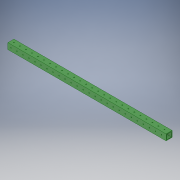
# Autodesk Inventor part: numbah 9
Saved by Autodesk Inventor 2018.2 (Build 222227000, 227)
## iProperties
Created: 2018-02-03
Part Number: numbah 9
Material: Generic
Document SubType Name: Modeling
Designer: matuch.michael
Density: 1 g/cm^3
Appearance: Smooth - Dark Forest Green
Author: matuch.michael
Autodesk Inventor part; units mm, degrees
ref_plane "YZ Plane" through (0, 0, 0) normal (1, 0, 0) x (0, 1, 0)
ref_plane "XZ Plane" through (0, 0, 0) normal (0, 1, 0) x (-1, 0, 0)
ref_plane "XY Plane" through (0, 0, 0) normal (0, 0, 1) x (1, 0, 0)
sketch "Sketch1" plane through (0, 0, 0) normal (0, 0, 1) x (1, 0, 0)
  line L0 (-12.5902, 5.4476) -> (654.49, 5.4476)
  line L1 (654.49, 5.4476) -> (654.49, -19.9524)
  line L2 (654.49, -19.9524) -> (-12.5902, -19.9524)
  line L3 (-12.5902, -19.9524) -> (-12.5902, 5.4476)
  point P0 (0, 0)
  dimension "d0" = 667.0802
  dimension "d1" = 25.4
  constraints: 8 end point, 2 parallel, 1 horizontal, 1 perpendicular
  measures "d0" distance of L1.end L2.end
  measures "d1" distance of L0.end L1.end
extrude "Extrusion1" add sketch "Sketch1" along normal blind 25.4
sketch "Sketch2" plane through (0, 0, 25.4) normal (0, 0, 1) x (1, 0, 0)
  circle A0 centre (0.1098, -7.2524) radius 1.9685
  line L0 (-12.5902, 5.4476) -> (-12.5902, -19.9524) projected
  line L1 (-12.5902, -19.9524) -> (654.49, -19.9524) projected
  circle A1 centre (25.5098, -7.2524) radius 1.9685
  circle A2 centre (50.9098, -7.2524) radius 1.9685
  circle A3 centre (76.3098, -7.2524) radius 1.9685
  circle A4 centre (101.7098, -7.2524) radius 1.9685
  circle A5 centre (127.1098, -7.2524) radius 1.9685
  circle A6 centre (152.5098, -7.2524) radius 1.9685
  circle A7 centre (177.9098, -7.2524) radius 1.9685
  circle A8 centre (203.3098, -7.2524) radius 1.9685
  circle A9 centre (228.7098, -7.2524) radius 1.9685
  circle A10 centre (254.1098, -7.2524) radius 1.9685
  circle A11 centre (279.5098, -7.2524) radius 1.9685
  circle A12 centre (304.9098, -7.2524) radius 1.9685
  circle A13 centre (330.3098, -7.2524) radius 1.9685
  circle A14 centre (355.7098, -7.2524) radius 1.9685
  circle A15 centre (381.1098, -7.2524) radius 1.9685
  circle A16 centre (406.5098, -7.2524) radius 1.9685
  circle A17 centre (431.9098, -7.2524) radius 1.9685
  circle A18 centre (457.3098, -7.2524) radius 1.9685
  circle A19 centre (482.7098, -7.2524) radius 1.9685
  circle A20 centre (508.1098, -7.2524) radius 1.9685
  circle A21 centre (533.5098, -7.2524) radius 1.9685
  circle A22 centre (558.9098, -7.2524) radius 1.9685
  circle A23 centre (584.3098, -7.2524) radius 1.9685
  circle A24 centre (609.7098, -7.2524) radius 1.9685
  circle A25 centre (635.1098, -7.2524) radius 1.9685
  circle A26 centre (635.1098, -7.2524) radius 1.9685
  circle A27 centre (660.5098, -7.2524) radius 1.9685
  circle A28 centre (685.9098, -7.2524) radius 1.9685
  point P0 (0, 0)
  dimension "d4" = 3.937
  dimension "d5" = 12.7
  dimension "d6" = 12.7
  dimension "d9" = 25.4
  dimension "d16" = 25.4
  constraints: 29 centre point, 2 horizontal, 56 other
  measures "d4" diameter of A0
  measures "d5" distance from line of L0 A0.centre
  measures "d6" distance from line of L1 A0.centre
  measures "d9" distance of A0.centre A1.centre
  measures "d16" distance of A24.centre A25.centre
sketch "Sketch4" plane through (-12.5902, 5.4476, 0) normal (0, 1, 0) x (1, 0, 0)
  circle A0 centre (12.7, -12.7) radius 1.9685
  line L0 (0, 0) -> (0, -25.4) projected
  line L1 (667.0802, -25.4) -> (0, -25.4) projected
  circle A1 centre (38.1, -12.7) radius 1.9685
  circle A2 centre (63.5, -12.7) radius 1.9685
  circle A3 centre (88.9, -12.7) radius 1.9685
  circle A4 centre (114.3, -12.7) radius 1.9685
  circle A5 centre (139.7, -12.7) radius 1.9685
  circle A6 centre (165.1, -12.7) radius 1.9685
  circle A7 centre (190.5, -12.7) radius 1.9685
  circle A8 centre (215.9, -12.7) radius 1.9685
  circle A9 centre (241.3, -12.7) radius 1.9685
  circle A10 centre (266.7, -12.7) radius 1.9685
  circle A11 centre (292.1, -12.7) radius 1.9685
  circle A12 centre (317.5, -12.7) radius 1.9685
  circle A13 centre (342.9, -12.7) radius 1.9685
  circle A14 centre (368.3, -12.7) radius 1.9685
  circle A15 centre (393.7, -12.7) radius 1.9685
  circle A16 centre (419.1, -12.7) radius 1.9685
  circle A17 centre (444.5, -12.7) radius 1.9685
  circle A18 centre (469.9, -12.7) radius 1.9685
  circle A19 centre (495.3, -12.7) radius 1.9685
  circle A20 centre (520.7, -12.7) radius 1.9685
  circle A21 centre (546.1, -12.7) radius 1.9685
  circle A22 centre (571.5, -12.7) radius 1.9685
  circle A23 centre (596.9, -12.7) radius 1.9685
  circle A24 centre (622.3, -12.7) radius 1.9685
  circle A25 centre (647.7, -12.7) radius 1.9685
  circle A26 centre (673.1, -12.7) radius 1.9685
  circle A27 centre (698.5, -12.7) radius 1.9685
  point P0 (12.5902, 0)
  dimension "d27" = 3.937
  dimension "d28" = 12.7
  dimension "d29" = 12.7
  dimension "d32" = 25.4
  constraints: 28 centre point, 1 horizontal, 54 other
  measures "d27" diameter of A0
  measures "d28" distance from line of L0 A0.centre
  measures "d29" distance from line of L1 A0.centre
  measures "d32" distance of A0.centre A1.centre
shell "Shell1" thickness 3.175 removed faces 2 at (654.49, -3.019, 8.4667) at (-12.5902, -11.4857, 16.9333)
extrude "Extrusion5" cut sketch "Sketch2" against normal blind 25.4
extrude "Extrusion6" cut sketch "Sketch4" against normal blind 25.4
body "Solid1"
